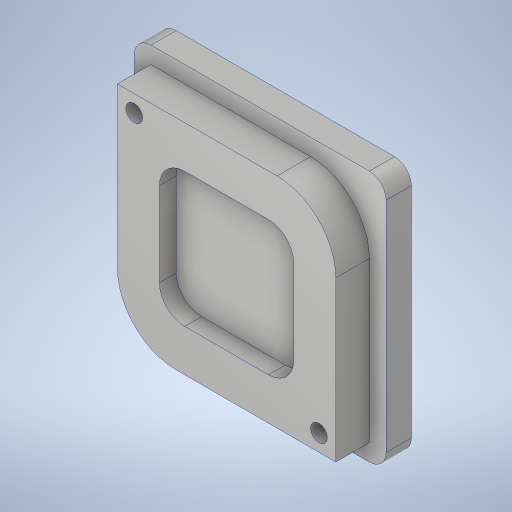
# Autodesk Inventor part: KUMAR_ACT6_L1
Saved by Autodesk Inventor 2024 (Build 280153000, 153)
## iProperties
Created: 2024-10-17
Part Number: KUMAR_ACT6_L1
Material: Aluminum 6061
Document SubType Name: Modeling
Designer: NK
Density: 2.7 g/cm^3
Appearance: Aluminum - Flat
Mass: 403.082 g
Surface Area: 290.728 cm^2
Volume: 149.29 cm^3
Author: NK
Autodesk Inventor part; units mm, degrees
ref_plane "YZ Plane" through (0, 0, 0) normal (1, 0, 0) x (0, 1, 0)
ref_plane "XZ Plane" through (0, 0, 0) normal (0, 1, 0) x (-1, 0, 0)
ref_plane "XY Plane" through (0, 0, 0) normal (0, 0, 1) x (1, 0, 0)
sketch "Sketch1" plane through (0, 0, 0) normal (0, 0, 1) x (1, 0, 0)
  line L0 (-47.625, 47.625) -> (47.625, 47.625)
  line L1 (47.625, 47.625) -> (47.625, -47.625)
  line L2 (47.625, -47.625) -> (-47.625, -47.625)
  line L3 (-47.625, -47.625) -> (-47.625, 47.625)
  line L4 (-47.625, 47.625) -> (47.625, -47.625) construction
  line L5 (47.625, 47.625) -> (-47.625, -47.625) construction
  point P0 (0, 0)
  dimension "d0" = 95.25
  dimension "d1" = 95.25
  constraints: 12 end point, 2 midpoint, 2 parallel, 1 horizontal, 1 perpendicular
  measures "d0" distance of L1.end L2.end
  measures "d1" distance of L0.end L1.end
extrude "Extrusion1" add sketch "Sketch1" along normal blind 9.525
sketch "Sketch2" plane through (0, 0, 9.525) normal (0, 0, 1) x (1, 0, 0)
  line L0 (41.275, -41.275) -> (-41.275, -41.275)
  line L1 (-41.275, -41.275) -> (-41.275, 41.275)
  line L2 (-41.275, 41.275) -> (41.275, 41.275)
  line L3 (41.275, 41.275) -> (41.275, -41.275)
  line L4 (41.275, -41.275) -> (-41.275, 41.275) construction
  line L5 (-41.275, -41.275) -> (41.275, 41.275) construction
  point P0 (0, 0)
  dimension "d4" = 82.55
  dimension "d5" = 82.55
  constraints: 12 end point, 2 midpoint, 2 parallel, 1 horizontal, 1 perpendicular
  measures "d4" distance of L1.end L2.end
  measures "d5" distance of L0.end L1.end
extrude "Extrusion2" add sketch "Sketch2" along normal blind 12.7
sketch "Sketch3" plane through (0, 0, 22.225) normal (0, 0, 1) x (1, 0, 0)
  line L0 (-25.4, -25.4) -> (25.4, -25.4)
  line L1 (25.4, -25.4) -> (25.4, 25.4)
  line L2 (25.4, 25.4) -> (-25.4, 25.4)
  line L3 (-25.4, 25.4) -> (-25.4, -25.4)
  line L4 (-25.4, -25.4) -> (25.4, 25.4) construction
  line L5 (25.4, -25.4) -> (-25.4, 25.4) construction
  point P0 (0, 0)
  dimension "d8" = 50.8
  dimension "d9" = 50.8
  constraints: 12 end point, 2 midpoint, 2 parallel, 1 horizontal, 1 perpendicular
  measures "d8" distance of L2.end L1.end
  measures "d9" distance of L1.end L0.end
extrude "Extrusion3" cut sketch "Sketch3" against normal blind 6.35
sketch "Sketch4" plane through (0, 0, 22.225) normal (0, 0, 1) x (1, 0, 0)
  line L0 (-41.275, 41.275) -> (-41.275, -41.275) projected
  line L1 (41.275, 41.275) -> (-41.275, 41.275) projected
  line L2 (-41.275, -41.275) -> (41.275, -41.275) projected
  line L3 (41.275, -41.275) -> (41.275, 41.275) projected
  point P0 (0, 0)
  point P1 (-34.925, 34.925)
  point P2 (34.925, -34.925)
  dimension "d19" = 6.35
  dimension "d20" = 6.35
  dimension "d21" = 6.35
  dimension "d22" = 6.35
  measures "d19" distance from line of L0 point (-34.925, 34.925)
  measures "d20" distance from line of L1 point (-34.925, 34.925)
  measures "d21" distance from line of L2 point (34.925, -34.925)
  measures "d22" distance from line of L3 point (34.925, -34.925)
hole "Hole1" at (-34.925, 34.925, 22.225) at (34.925, -34.925, 22.225) direction (0, 0, -1) diameter 6.35 end through all
sketch "Sketch5" plane through (0, 0, 0) normal (0, 0, -1) x (-1, 0, 0)
  point P0 (0, 0)
  point P1 (-28.575, 28.575)
  point P2 (28.575, 28.575)
  point P3 (28.575, -28.575)
  point P4 (-28.575, -28.575)
  dimension "d37" = 57.15
  dimension "d38" = 28.575
  dimension "d39" = 57.15
  dimension "d40" = 28.575
  dimension "d41" = 57.15
  dimension "d42" = 57.15
  dimension "d43" = 28.575
  dimension "d44" = 28.575
  measures "d37" distance of point (-28.575, 28.575) point (28.575, 28.575)
  measures "d38" horizontal distance of point (0, 0) point (28.575, 28.575)
  measures "d39" distance of point (28.575, -28.575) point (-28.575, -28.575)
  measures "d40" horizontal distance of point (28.575, -28.575) point (0, 0)
  measures "d41" distance of point (-28.575, 28.575) point (-28.575, -28.575)
  measures "d42" distance of point (28.575, 28.575) point (28.575, -28.575)
  measures "d43" horizontal distance of point (0, 0) point (28.575, -28.575)
  measures "d44" horizontal distance of point (-28.575, 28.575) point (0, 0)
hole "Hole2" at (28.575, 28.575, 0) at (-28.575, 28.575, 0) at (-28.575, -28.575, 0) at (28.575, -28.575, 0) direction (0, 0, 1) diameter 7.9502 depth 15.875 tip angle 118 countersink diameter 9.525 countersink angle 82
fillet "Fillet1" radius 6.35 4 edges at (47.625, -47.625, 4.7625) (-47.625, -47.625, 4.7625) (47.625, 47.625, 4.7625) (-47.625, 47.625, 4.7625)
fillet "Fillet3" radius 22.225 2 edges at (41.275, 41.275, 15.875) (-41.275, -41.275, 15.875)
fillet "Fillet4" radius 9.525 4 edges at (-25.4, 25.4, 19.05) (-25.4, -25.4, 19.05) (25.4, 25.4, 19.05) (25.4, -25.4, 19.05)
thread "Thread1" size "3/8-16 UNC" class "2B" standard "ANSI Unified Screw Threads" full length
thread "Thread2" size "3/8-16 UNC" class "2B" standard "ANSI Unified Screw Threads" full length
thread "Thread3" size "3/8-16 UNC" class "2B" standard "ANSI Unified Screw Threads" full length
thread "Thread4" size "3/8-16 UNC" class "2B" standard "ANSI Unified Screw Threads" full length
body "Solid1"
